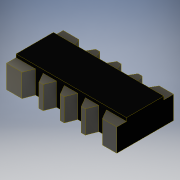
# Autodesk Inventor part: 746SeriesR
Saved by Autodesk Inventor 2016 (Build 200138000, 138)
## iProperties
Created: 2017-03-03
Part Number: 746SeriesR
Material: Generic
Document SubType Name: Modeling
Designer: jfixelle
Density: 1 g/cm^3
Appearance: Silver
Author: jfixelle
Autodesk Inventor part; units mm, degrees
ref_plane "YZ Plane" through (0, 0, 0) normal (1, 0, 0) x (0, 1, 0)
ref_plane "XZ Plane" through (0, 0, 0) normal (0, 1, 0) x (-1, 0, 0)
ref_plane "XY Plane" through (0, 0, 0) normal (0, 0, 1) x (1, 0, 0)
sketch "Sketch1" plane through (0, 0, 0) normal (0, 1, 0) x (-1, 0, 0)
  line L0 (1.7, 0.875) -> (-1.7, 0.875)
  line L1 (-1.7, 0.875) -> (-1.7, -0.875)
  line L2 (-1.7, -0.875) -> (1.7, -0.875)
  line L3 (1.7, -0.875) -> (1.7, 0.875)
  point P0 (0, 0)
  dimension "d0" = 1.75
  dimension "d1" = 0.875
  dimension "d2" = 1.7
  dimension "d3" = 3.4
  constraints: 8 end point, 2 parallel, 1 horizontal, 1 perpendicular
  measures "d0" distance of L2.end L0.start
  measures "d1" distance from line of point (0, 0) L2
  measures "d2" distance from line of point (0, 0) L3
  measures "d3" distance of L1.end L2.end
extrude "Extrusion1" add sketch "Sketch1" along normal blind 0.7
sketch "Sketch3" plane through (0, 0.7, 0) normal (0, 1, 0) x (1, 0, 0)
  line L0 (1.7, -0.875) -> (1.7, -0.575)
  line L1 (1.7, -0.875) -> (1.7, 0.875) projected
  line L2 (-1.7, -0.875) -> (1.7, -0.875) projected
  line L3 (0.6665, -0.875) -> (0.6665, -0.575)
  line L4 (1.4815, -0.875) -> (1.4815, -0.745)
  line L5 (1.0816, -0.575) -> (0.8481, -0.575)
  line L6 (1.2548, -0.875) -> (0.7314, -0.875)
  line L7 (0.7314, -0.875) -> (0.8481, -0.575)
  line L8 (1.0816, -0.575) -> (1.2548, -0.875)
  point P0 (0, 0)
  dimension "d9" = 0
  dimension "d24" = 0.2185
  dimension "d25" = 120
  dimension "d26" = 111.251
  dimension "d27" = 0.2335
  dimension "d29" = 68.749
  constraints: 14 end point, 2 point on line
  measures "d9" distance between parallel lines of L1 L0
  measures "d24" distance between parallel lines of L0 L4
  measures "d25" angle of L5 L8
  measures "d26" angle of L5 L7
  measures "d27" distance of L5.start L5.end
  measures "d29" angle of L2 L7
extrude "Extrusion2" cut sketch "Sketch3" against normal blind 0.7
pattern_linear "Rectangular Pattern1" count 4 spacing 0.65 along (-1, 0, 0) of "Extrusion2"
mirror "Mirror1" about plane through (0, 0, 0) normal (0, 0, 1) of "Extrusion2", "Rectangular Pattern1"
sketch "Sketch4" plane through (0, 0.7, 0) normal (0, 1, 0) x (1, 0, 0)
  line L0 (1.7, -0.875) -> (1.7, 0.875) projected
  line L1 (-1.7, 0.875) -> (-1.7, -0.875) projected
  line L2 (1.7, 0.575) -> (-1.7, 0.575)
  line L3 (-1.7, 0.575) -> (-1.7, -0.575)
  line L4 (-1.7, -0.575) -> (1.7, -0.575)
  line L5 (1.7, -0.575) -> (1.7, 0.575)
  point P0 (0, 0)
  constraints: 8 end point, 2 parallel, 2 point on line, 1 horizontal, 1 perpendicular
extrude "Extrusion3" add sketch "Sketch4" along normal blind 0.1
body "Solid1"
